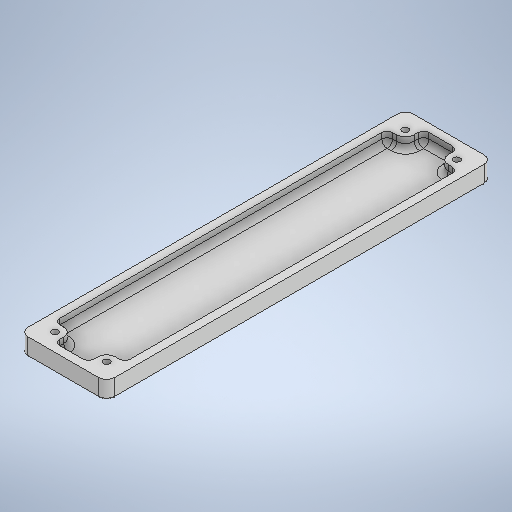
# Autodesk Inventor part: Lower_Housing
Saved by Autodesk Inventor 2025 (Build 290162010, 162A)
## iProperties
Created: 2025-09-30
Part Number: Lower_Housing
Material: Genérico
Document SubType Name: Modeling
Designer: João Vitor
Density: 1 g/cm^3
Appearance: Padrão
Author: João Vitor
Autodesk Inventor part; units mm, degrees
ref_plane "YZ Plane" through (0, 0, 0) normal (1, 0, 0) x (0, 1, 0)
ref_plane "XZ Plane" through (0, 0, 0) normal (0, 1, 0) x (-1, 0, 0)
ref_plane "XY Plane" through (0, 0, 0) normal (0, 0, 1) x (1, 0, 0)
sketch "Esboço1" plane through (0, 0, 0) normal (0, 1, 0) x (-1, 0, 0)
  line L0 (-10, 68) -> (10, 68)
  line L1 (13, 65) -> (13, -65)
  line L2 (10, -68) -> (-10, -68)
  line L3 (-13, -65) -> (-13, 65)
  line L4 (-13, 68) -> (13, -68) construction
  line L5 (13, 68) -> (-13, -68) construction
  circle A0 centre (9.5, 64.5) radius 1.2
  circle A1 centre (-9.5, 64.5) radius 1.2
  circle A2 centre (-9.5, -64.5) radius 1.2
  circle A3 centre (9.5, -64.5) radius 1.2
  line L6 (-13, 71) -> (13, 71)
  line L7 (16, 68) -> (16, -68)
  line L8 (13, -71) -> (-13, -71)
  line L9 (-16, -68) -> (-16, 68)
  line L10 (-16, 71) -> (16, -71) construction
  line L11 (16, 71) -> (-16, -71) construction
  arc A4 (-13, 71) -> (-16, 68) centre (-13, 68) ccw
  arc A5 (-10, 68) -> (-13, 65) centre (-10, 65) ccw
  arc A6 (13, 65) -> (10, 68) centre (10, 65) ccw
  arc A7 (16, 68) -> (13, 71) centre (13, 68) ccw
  arc A8 (13, -71) -> (16, -68) centre (13, -68) ccw
  arc A9 (10, -68) -> (13, -65) centre (10, -65) ccw
  arc A10 (-13, -65) -> (-10, -68) centre (-10, -65) ccw
  arc A11 (-16, -68) -> (-13, -71) centre (-13, -68) ccw
  circle A12 centre (-9.5, 64.5) radius 3.2
  circle A13 centre (9.5, 64.5) radius 3.2
  circle A14 centre (9.5, -64.5) radius 3.2
  circle A15 centre (-9.5, -64.5) radius 3.2
  line L12 (-9.5, 61.3) -> (-13, 61.3)
  line L13 (-6.3, 64.5) -> (-6.3, 68)
  line L14 (6.3, 64.5) -> (6.3, 68)
  line L15 (9.5, 61.3) -> (13, 61.3)
  line L16 (-9.5, -61.3) -> (-13, -61.3)
  line L17 (-6.3, -64.5) -> (-6.3, -68)
  line L18 (6.3, -64.5) -> (6.3, -68)
  line L19 (9.5, -61.3) -> (13, -61.3)
  point P0 (0, 0)
  dimension "d0" = 136
  dimension "d1" = 26
  dimension "d2" = 3.5
  dimension "d3" = 3.5
  dimension "d4" = 3.5
  dimension "d5" = 3.5
  dimension "d6" = 2.4
  dimension "d7" = 3
  dimension "d8" = 3
  dimension "d9" = 3
  dimension "d12" = 2
  dimension "d13" = 2
  dimension "d14" = 2
  dimension "d15" = 2
  constraints: 40 end point, 26 point on line, 24 point on circle, 23 tangent, 16 centre point, 10 equal radius, 9 perpendicular, 4 coincident, 4 midpoint, 4 parallel, 2 horizontal, 2 horizontal alignment, 2 vertical alignment
  measures "d0" distance between parallel lines of L2 L0
  measures "d1" distance between parallel lines of L1 L3
  measures "d2" distance from line of L3 A1.centre
  measures "d3" distance from line of L0 A1.centre
  measures "d4" distance from line of L2 A3.centre
  measures "d5" distance from line of L1 A3.centre
  measures "d6" diameter of A2
  measures "d7" distance between parallel lines of L7 L1
  measures "d8" distance between parallel lines of L8 L2
  measures "d9" radius of A4
  measures "d12" radial gap between concentric circles of A12 A1
  measures "d13" radial gap between concentric circles of A13 A0
  measures "d14" radial gap between concentric circles of A15 A2
  measures "d15" radial gap between concentric circles of A14 A3
extrude "Extrusão1" add sketch "Esboço1" along normal blind 2.4 contours L0 L13 A12 L12 L3 A5 | L0 L14 A13 L15 L1 L19 A14 L18 L2 L17 A15 L16 L3 L12 A12 L13 | L0 A6 L1 L15 A13 L14 | A12 | A13 | L16 A15 L17 L2 A10 L3 | A15 | L1 A9 L2 L18 A14 L19 | A14 | A0 | A1 | A2 | A3
extrude "Extrusão2" add sketch "Esboço1" along normal blind 6.5 contours L0 L13 A12 L12 L3 A5 | L0 A6 L1 L15 A13 L14 | A12 | A13 | L16 A15 L17 L2 A10 L3 | A15 | L1 A9 L2 L18 A14 L19 | A14
extrude "Extrusão3" add sketch "Esboço1" along normal blind 6.5 contours L6 A7 L7 A8 L8 A11 L9 A4
fillet "Arredondamento1" radius 0.5 8 edges at (15.1213, 0, -70.1213) (0, 0, -71) (-15.1213, 0, -70.1213) (-16, 0, 0) (-15.1213, 0, 70.1213) (0, 0, 71) (15.1213, 0, 70.1213) (16, 0, 0)
fillet "Arredondamento2" radius 2 16 edges at (6.3, 2.4, -66.25) (11.25, 2.4, -61.3) (7.2373, 2.4, -62.2373) (0, 2.4, -68) (-7.2373, 2.4, -62.2373) (-6.3, 2.4, -66.25) (-11.25, 2.4, -61.3) (-13, 2.4, 0) (13, 2.4, 0) (11.25, 2.4, 61.3) (6.3, 2.4, 66.25) (7.2373, 2.4, 62.2373) (0, 2.4, 68) (-6.3, 2.4, 66.25) (-11.25, 2.4, 61.3) (-7.2373, 2.4, 62.2373)
fillet "Arredondamento3" radius 2 16 edges at (13, 5.45, 61.3) (12.4142, 2.9858, 60.7142) (6.3, 5.45, 68) (5.7142, 2.9858, 67.4142) (-12.4142, 2.9858, 60.7142) (-13, 5.45, 61.3) (-6.3, 5.45, 68) (-5.7142, 2.9858, 67.4142) (-12.4142, 2.9858, -60.7142) (-13, 5.45, -61.3) (-6.3, 5.45, -68) (-5.7142, 2.9858, -67.4142) (13, 5.45, -61.3) (12.4142, 2.9858, -60.7142) (6.3, 5.45, -68) (5.7142, 2.9858, -67.4142)
equation "\"d10\" = d6"
